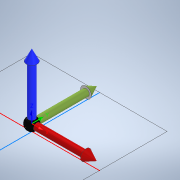
# Autodesk Inventor part: 0_Sistemariferimento
Saved by Autodesk Inventor 2020.2 (Build 242310000, 310)
## iProperties
Created: 2020-01-23
Part Number: 0_Sistemariferimento
Material: Generico
Document SubType Name: Modeling
Designer: socci
Density: 1 g/cm^3
Appearance: Default
Author: socci
Autodesk Inventor part; units mm, degrees
ref_plane "YZ Plane" through (0, 0, 0) normal (1, 0, 0) x (0, 1, 0)
ref_plane "XZ Plane" through (0, 0, 0) normal (0, 1, 0) x (-1, 0, 0)
ref_plane "XY Plane" through (0, 0, 0) normal (0, 0, 1) x (1, 0, 0)
sketch "Schizzo1" plane through (0, 0, 0) normal (0, 1, 0) x (-1, 0, 0)
  line L0 (1.5, 0) -> (-1.5, 0)
  arc A0 (1.5, 0) -> (-1.5, 0) centre (0, 0) ccw
  dimension "d11" = 3
  constraints: 2 coincident, 2 end point, 2 point on circle, 1 centre point, 1 horizontal, 1 midpoint
  measures "d11" distance of L0.start L0.end
revolve "Rivoluzione1" add sketch "Schizzo1" angle 360 about axis through (-1.5, 0, 0) along (1, 0, 0)
sketch "Schizzo3" plane through (0, 0, 0) normal (0, 0, -1) x (0, 1, 0)
  circle A0 centre (0, 0) radius 5
  dimension "d19" = 10
  constraints: 1 centre point, 1 coincident
  measures "d19" diameter of A0
extrude "Estrusione2" add sketch "Schizzo3" along normal blind 80
sketch "Schizzo4" plane through (0, 0, 0) normal (1, 0, 0) x (0, 0, -1)
  circle A0 centre (0, 0) radius 5
  dimension "d22" = 10
  constraints: 1 centre point, 1 coincident
  measures "d22" diameter of A0
extrude "Estrusione3" add sketch "Schizzo4" along normal blind 80
sketch "Schizzo5" plane through (0, 0, 0) normal (0, 1, 0) x (1, 0, 0)
  line L0 (0, -5) -> (0, 0) projected
  circle A0 centre (0, 0) radius 5
  dimension "d25" = 10
  constraints: 1 centre point, 1 coincident
  measures "d25" diameter of A0
extrude "Estrusione4" add sketch "Schizzo5" along normal blind 80
sketch "Schizzo6" plane through (0, 0, 0) normal (1, 0, 0) x (0, 0, -1)
  line L0 (0, -9) -> (0, 9)
  line L1 (0, 0) -> (-5, 0) projected
  arc A0 (0, -9) -> (0, 9) centre (0, 0) ccw
  dimension "d28" = 18
  constraints: 2 coincident, 2 end point, 2 point on circle, 1 centre point, 1 midpoint, 1 vertical
  measures "d28" distance of L0.start L0.end
revolve "Rivoluzione3" add sketch "Schizzo6" angle 360 about axis through (0, -9, 0) along (0, 1, 0)
sketch "Schizzo7" plane through (0, 0, 0) normal (0, 0, -1) x (0, 1, 0)
  line L0 (7.4833, -5) -> (7.4833, 5) projected
  line L1 (80, -5) -> (80, 5) projected
  line L2 (5, 7.4833) -> (-5, 7.4833) projected
  line L3 (5, 80) -> (-5, 80) projected
  line L4 (0, 0) -> (80, 0)
  line L5 (80, 0) -> (80, 8)
  line L6 (80, -5) -> (80, 5) projected
  line L7 (80, 0) -> (88, 0) construction
  line L8 (80, 0) -> (96, 0)
  line L9 (80, 0) -> (96, 0) construction
  line L10 (96, 0) -> (80, 8)
  point P0 (96, 0)
  dimension "d30" = 8
  dimension "d31" = 90
  dimension "d32" = 16
  dimension "d33" = 0
  constraints: 12 end point, 2 collinear, 2 equal length, 2 horizontal, 1 midpoint
  measures "d30" distance of L4.end L5.end
  measures "d31" angle of L7 L5
  measures "d32" distance of L4.end L8.end
  measures "d33" distance between parallel lines of L8 L9
revolve "Rivoluzione4" add sketch "Schizzo7" angle 360 about axis through (0, 80, 0) along (0, 1, 0)
sketch "Schizzo8" plane through (0, 0, 0) normal (1, 0, 0) x (0, 0, -1)
  line L0 (0, 0) -> (80, 0)
  line L1 (7.4833, -5) -> (7.4833, 5) projected
  line L2 (80, -5) -> (80, 5) projected
  line L3 (80, 0) -> (80, 8)
  line L4 (80, -5) -> (80, 5) projected
  line L5 (80, 0) -> (88, 0) construction
  line L6 (80, 0) -> (96, 0)
  line L7 (80, 0) -> (96, 0) construction
  line L8 (96, 0) -> (80, 8)
  dimension "d35" = 8
  dimension "d36" = 90
  dimension "d37" = 16
  dimension "d38" = 0
  constraints: 12 end point, 2 collinear, 2 equal length, 2 horizontal, 1 coincident, 1 midpoint
  measures "d35" distance of L0.end L3.end
  measures "d36" angle of L5 L3
  measures "d37" distance of L0.end L6.end
  measures "d38" distance between parallel lines of L6 L7
revolve "Rivoluzione5" add sketch "Schizzo8" angle 360 about axis through (0, 0, -80) along (0, 0, -1)
sketch "Schizzo9" plane through (0, 0, 0) normal (0, 0, -1) x (0, 1, 0)
  line L0 (5, 7.4833) -> (-5, 7.4833) projected
  line L1 (5, 80) -> (-5, 80) projected
  circle A0 centre (0, 0) radius 8 projected
  line L2 (0, 0) -> (0, 80)
  line L3 (0, 80) -> (8, 80)
  line L4 (5, 80) -> (-5, 80) projected
  line L5 (0, 80) -> (8, 80) construction
  line L6 (0, 80) -> (0, 96)
  line L7 (0, 80) -> (16, 80) construction
  line L8 (0, 96) -> (8, 80)
  dimension "d40" = 8
  dimension "d41" = 0
  dimension "d42" = 16
  dimension "d43" = 90
  constraints: 12 end point, 2 equal length, 2 horizontal, 1 coincident, 1 collinear, 1 midpoint, 1 perpendicular
  measures "d40" distance of L2.end L3.end
  measures "d41" distance between parallel lines of L3 L5
  measures "d42" distance of L2.end L6.end
  measures "d43" angle of L7 L6
revolve "Rivoluzione6" add sketch "Schizzo9" angle 360 about axis through (80, 0, 0) along (1, 0, 0) contours L1 L6 L8 L3
fillet "Raccordo1" radius 3 1 edges at (0, -5, -80)
fillet "Raccordo2" radius 3 1 edges at (-5, 80, 0)
fillet "Raccordo3" radius 3 1 edges at (80, 0, 5)
ref_plane "PianoY" through (0, 0, -96) normal (0, 0, -1) x (-1, 0, 0)
ref_plane "PianoX" through (96, 0, 0) normal (-1, 0, 0) x (0, -1, 0)
ref_plane "PianoZ" through (0, 96, 0) normal (0, 1, 0) x (-1, 0, 0)
